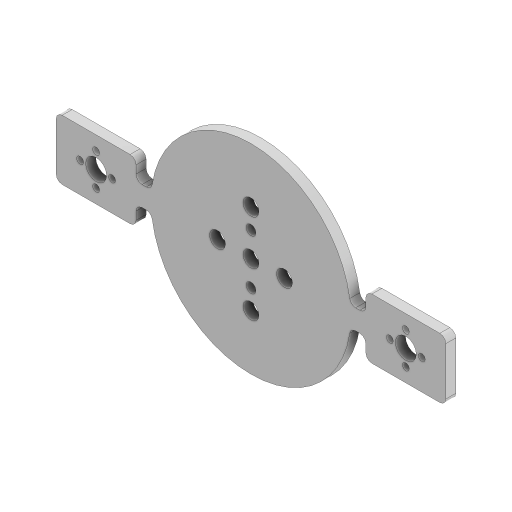
# Autodesk Inventor part: TAPA QUE DESPLAZA CON TORNILLOS
Saved by Autodesk Inventor 2024 (Build 280153000, 153)
## iProperties
Created: 2024-05-26
Part Number: TAPA QUE DESPLAZA CON TORNILLOS
Material: Generic
Document SubType Name: Modeling
Designer: Jhuliams
Density: 1 g/cm^3
Appearance: Default
Author: Jhuliams
Autodesk Inventor part; units mm, degrees
ref_plane "YZ Plane" through (0, 0, 0) normal (1, 0, 0) x (0, 1, 0)
ref_plane "XZ Plane" through (0, 0, 0) normal (0, 1, 0) x (-1, 0, 0)
ref_plane "XY Plane" through (0, 0, 0) normal (0, 0, 1) x (1, 0, 0)
sketch "Sketch1" plane through (0, 0, 0) normal (0, 0, 1) x (1, 0, 0)
  circle A0 centre (0, 0) radius 50
  line L0 (0, 0) -> (0, 20) construction
  line L1 (2.5, 15) -> (97.5, 15)
  line L2 (97.5, 15) -> (97.5, -15)
  line L3 (97.5, -15) -> (2.5, -15)
  line L4 (2.5, -15) -> (2.5, 15)
  line L5 (2.5, 15) -> (97.5, -15) construction
  line L6 (97.5, 15) -> (2.5, -15) construction
  line L7 (42.5, 5) -> (57.5, 5)
  line L8 (57.5, 5) -> (57.5, -5)
  line L9 (57.5, -5) -> (42.5, -5)
  line L10 (42.5, -5) -> (42.5, 5)
  line L11 (42.5, 5) -> (57.5, -5) construction
  line L12 (57.5, 5) -> (42.5, -5) construction
  line L13 (57.5, 5) -> (57.5, 15)
  line L14 (57.5, -5) -> (57.5, -15)
  line L15 (-2.5, 15) -> (-97.5, 15)
  line L16 (-97.5, 15) -> (-97.5, -15)
  line L17 (-97.5, -15) -> (-2.5, -15)
  line L18 (-2.5, -15) -> (-2.5, 15)
  line L19 (-2.5, 15) -> (-97.5, -15) construction
  line L20 (-97.5, 15) -> (-2.5, -15) construction
  line L21 (-42.5, 5) -> (-57.5, 5)
  line L22 (-57.5, 5) -> (-57.5, -5)
  line L23 (-57.5, -5) -> (-42.5, -5)
  line L24 (-42.5, -5) -> (-42.5, 5)
  line L25 (-42.5, 5) -> (-57.5, -5) construction
  line L26 (-57.5, 5) -> (-42.5, -5) construction
  line L27 (-57.5, 5) -> (-57.5, 15)
  line L28 (-57.5, -5) -> (-57.5, -15)
  point P0 (50, 0)
  point P1 (50, 0)
  point P2 (-50, 0)
  point P3 (-50, 0)
  point P4 (49.7494, 5)
  point P5 (49.7494, -5)
  point P6 (-49.7494, -5)
  point P7 (-49.7494, 5)
  dimension "d0" = 100
  dimension "d3" = 20
  dimension "d17" = 95
  dimension "d18" = 30
  dimension "d19" = 15
  dimension "d20" = 10
  constraints: 58 end point, 12 symmetric about line, 5 midpoint, 4 parallel, 4 perpendicular, 4 point on line, 2 horizontal, 1 coincident, 1 vertical, 3 other
  measures "d3" distance of L0.start L0.end
  measures "d17" distance of L2.end L3.end
  measures "d18" distance of L1.end L2.end
  measures "d19" distance of L8.end L9.end
  measures "d20" distance of L7.end L8.end
extrude "Extrusion1" add sketch "Sketch1" along normal blind 5 contours A0 L9 L10 L7 | A0 L7 L8 L9 | L7 L10 L9 A0 L3 L4 L1 | L1 L4 L3 A0 L17 L18 L15 | L13 L1 L2 L3 L14 L8 | L15 L18 L17 A0 L23 L24 L21 | L21 L24 L23 A0 | A0 L23 L22 L21 | L27 L22 L28 L17 L16 L15
sketch "Sketch2" plane through (0, 0, 5) normal (0, 0, 1) x (1, 0, 0)
  line L0 (0, 0) -> (-77.5, 0) construction
  circle A0 centre (-77.5, 0) radius 5.25
  line L1 (0, 0) -> (0, 20) construction
  circle A1 centre (-77.5, 0) radius 8
  circle A2 centre (-69.5, 0) radius 1.75
  circle A3 centre (-77.5, 8) radius 1.75
  circle A4 centre (-85.5, 0) radius 1.75
  circle A5 centre (-77.5, -8) radius 1.75
  circle A6 centre (77.5, 0) radius 5.25
  circle A7 centre (77.5, 0) radius 8
  circle A8 centre (69.5, 0) radius 1.75
  circle A9 centre (77.5, 8) radius 1.75
  circle A10 centre (85.5, 0) radius 1.75
  circle A11 centre (77.5, -8) radius 1.75
  dimension "d26" = 16
  dimension "d6" = 77.5
  dimension "d7" = 10.5
  dimension "d8" = 20
  dimension "d27" = 3.5
  dimension "d30" = 360
  constraints: 10 centre point, 7 symmetric about line, 6 coincident, 4 end point, 2 horizontal alignment, 2 point on line, 2 vertical, 1 horizontal, 18 other
  measures "d6" distance of L0.start L0.end
  measures "d7" diameter of A0
  measures "d8" distance of L0.start L1.end
  measures "d27" diameter of A2
extrude "Extrusion2" cut sketch "Sketch2" against normal blind 7 contours A0 | A1 A2 | A1 A2 | A3 A1 | A1 A3 | A5 A1 | A1 A5 | A4 A1 | A1 A4 | A6 | A7 A10 | A7 A10 | A9 A7 | A7 A9 | A11 A7 | A7 A11 | A8 A7 | A7 A8
fillet "Fillet1" radius 3 16 edges at (-57.5, 5, 2.5) (-57.5, 15, 2.5) (-49.7494, 5, 2.5) (-57.5, -5, 2.5) (-57.5, -15, 2.5) (-49.7494, -5, 2.5) (-97.5, -15, 2.5) (-97.5, 15, 2.5) (97.5, 15, 2.5) (97.5, -15, 2.5) (57.5, -15, 2.5) (57.5, 15, 2.5) (57.5, -5, 2.5) (57.5, 5, 2.5) (49.7494, 5, 2.5) (49.7494, -5, 2.5)
sketch "Sketch4" plane through (0, 0, 5) normal (0, 0, 1) x (1, 0, 0)
  line L0 (-17.5, 5) -> (17.5, 5)
  line L1 (17.5, 5) -> (17.5, -5)
  line L2 (17.5, -5) -> (-17.5, -5)
  line L3 (-17.5, -5) -> (-17.5, 5)
  line L4 (-17.5, 5) -> (17.5, -5) construction
  line L5 (17.5, 5) -> (-17.5, -5) construction
  circle A0 centre (0, -5) radius 17.5
  circle A1 centre (0, 5) radius 17.5
  circle A2 centre (0, -22.5) radius 4
  circle A3 centre (0, 22.5) radius 4
  circle A4 centre (0, 0) radius 4
  circle A5 centre (16.7705, 0) radius 4
  circle A6 centre (-16.7705, 0) radius 4
  circle A7 centre (0, -12.5) radius 2.5
  circle A8 centre (0, 12.5) radius 2.5
  dimension "d32" = 35
  dimension "d33" = 10
  dimension "d34" = 35
  dimension "d35" = 35
  dimension "d36" = 8
  dimension "d37" = 8
  dimension "d38" = 8
  dimension "d39" = 8
  dimension "d40" = 8
  dimension "d41" = 5
  dimension "d42" = 5
  constraints: 12 end point, 9 centre point, 8 point on circle, 2 midpoint, 2 parallel, 1 coincident, 1 horizontal, 1 perpendicular
  measures "d32" distance of L1.end L2.end
  measures "d33" distance of L0.end L1.end
  measures "d34" diameter of A0
  measures "d35" diameter of A1
  measures "d36" diameter of A2
  measures "d37" diameter of A3
  measures "d38" diameter of A4
  measures "d39" diameter of A5
  measures "d40" diameter of A6
  measures "d41" diameter of A7
  measures "d42" diameter of A8
extrude "Extrusion3" cut sketch "Sketch4" against normal blind 10 contours A6 A1 A0 L3 | L3 A6 | A3 A1 | A1 A3 | A6 A0 A1 | A8 A0 | A0 A8 | A6 A1 A0 | A1 A6 A0 | A5 A1 A0 | A0 A1 A5 | A5 L1 | L1 A5 A0 A1 | A0 A5 A1 | A2 A0 | A0 A2 | A7 A1 | A1 A7 | A4
body "Solid1"
